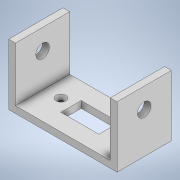
# Autodesk Inventor part: base and 1st arm link
Saved by Autodesk Inventor 2022 (Build 260153000, 153)
## iProperties
Created: 2021-06-29
Part Number: base and 1st arm link
Material: Generic
Document SubType Name: Modeling
Designer: USER
Density: 1 g/cm^3
Appearance: Default
Author: USER
Autodesk Inventor part; units mm, degrees
ref_plane "YZ Plane" through (0, 0, 0) normal (1, 0, 0) x (0, 1, 0)
ref_plane "XZ Plane" through (0, 0, 0) normal (0, 1, 0) x (-1, 0, 0)
ref_plane "XY Plane" through (0, 0, 0) normal (0, 0, 1) x (1, 0, 0)
sketch "Sketch1" plane through (0, 0, 0) normal (0, 0, 1) x (1, 0, 0)
  line L0 (0, 0) -> (0, 45)
  line L1 (0, 45) -> (5, 45)
  line L2 (5, 45) -> (5, 5)
  line L3 (5, 5) -> (75, 5)
  line L4 (75, 5) -> (75, 45)
  line L5 (75, 45) -> (80, 45)
  line L6 (80, 45) -> (80, 0)
  line L7 (80, 0) -> (0, 0)
  dimension "d0" = 45
  dimension "d1" = 5
  dimension "d2" = 40
  dimension "d3" = 70
  dimension "d4" = 40
  dimension "d5" = 5
  dimension "d6" = 45
  constraints: 16 end point, 4 perpendicular, 2 point on line, 1 vertical
  measures "d0" distance of L0.start L0.end
  measures "d1" distance of L0.end L1.end
  measures "d2" distance of L1.end L2.end
  measures "d3" distance of L2.end L3.end
  measures "d4" distance of L3.end L4.end
  measures "d5" distance of L4.end L5.end
  measures "d6" distance of L5.end L6.end
extrude "Extrusion1" add sketch "Sketch1" along normal blind 40
sketch "Sketch2" plane through (80, 0, 0) normal (1, 0, 0) x (0, 0, -1)
  circle A0 centre (-20, 30) radius 5
  line L0 (0, 45) -> (-40, 45) projected
  line L1 (0, 0) -> (0, 45) projected
  dimension "d9" = 10
  dimension "d10" = 15
  dimension "d11" = 20
  constraints: 1 centre point
  measures "d9" diameter of A0
  measures "d10" distance from line of L0 A0.centre
  measures "d11" distance from line of L1 A0.centre
extrude "Extrusion2" cut sketch "Sketch2" against normal through all
sketch "Sketch3" plane through (5, 5, 0) normal (0, 1, 0) x (1, 0, 0)
  line L0 (21, -12.5) -> (49, -12.5)
  line L1 (49, -12.5) -> (49, -27.5)
  line L2 (49, -27.5) -> (21, -27.5)
  line L3 (21, -27.5) -> (21, -12.5)
  line L4 (21, -12.5) -> (49, -27.5) construction
  line L5 (49, -12.5) -> (21, -27.5) construction
  line L6 (70, 0) -> (0, 0) projected
  line L7 (0, 0) -> (0, -40) projected
  point P0 (-5, 0)
  point P1 (35, -20)
  dimension "d14" = 28
  dimension "d15" = 15
  dimension "d16" = 20
  dimension "d17" = 35
  constraints: 12 end point, 2 midpoint, 2 parallel, 1 horizontal, 1 perpendicular
  measures "d14" distance of L1.end L2.end
  measures "d15" distance of L0.end L1.end
  measures "d16" distance from line of L6 point (35, -20)
  measures "d17" distance from line of L7 point (35, -20)
extrude "Extrusion3" cut sketch "Sketch3" against normal blind 10
sketch "Sketch4" plane through (5, 5, 0) normal (0, 1, 0) x (1, 0, 0)
  circle A0 centre (12, -18.4275) radius 3.625
  circle A1 centre (58, -18.4275) radius 3.625
  line L0 (21, -27.5) -> (21, -12.5) projected
  line L1 (49, -12.5) -> (49, -27.5) projected
  point P0 (-5, 0)
  dimension "d20" = 7.25
  dimension "d21" = 7.25
  dimension "d22" = 9
  dimension "d23" = 9
  constraints: 2 centre point
  measures "d20" diameter of A0
  measures "d21" diameter of A1
  measures "d22" distance from line of L0 A0.centre
  measures "d23" distance from line of L1 A1.centre
extrude "Extrusion4" cut sketch "Sketch4" against normal blind 2.1735 draft -45
sketch "Sketch5" plane through (17, 2.8265, 18.4275) normal (0, 1, 0) x (1, 0, 0)
  circle A0 centre (0, 0) radius 1.4515
  circle A1 centre (46, 0) radius 1.4515
  line L0 (37, 5.9275) -> (37, -9.0725) projected
  point P0 (-17, 18.4275)
  dimension "d26" = 2.903
  dimension "d27" = 9
  constraints: 2 centre point
  measures "d26" diameter of A1
  measures "d27" distance from line of L0 A1.centre
extrude "Extrusion5" cut sketch "Sketch5" against normal through all
body "Solid1"
